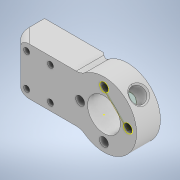
# Autodesk Inventor part: armtip_1
Saved by Autodesk Inventor 2020 (Build 240168000, 168)
## iProperties
Created: 2019-10-15
Part Number: armtip_1
Material: Generic
Document SubType Name: Modeling
Designer: psrob
Density: 1 g/cm^3
Appearance: Default
Author: psrob
Autodesk Inventor part; units mm, degrees
ref_plane "YZ Plane" through (0, 0, 0) normal (1, 0, 0) x (0, 1, 0)
ref_plane "XZ Plane" through (0, 0, 0) normal (0, 1, 0) x (-1, 0, 0)
ref_plane "XY Plane" through (0, 0, 0) normal (0, 0, 1) x (1, 0, 0)
sketch "Sketch1" plane through (0, 0, 0) normal (0, 0, 1) x (1, 0, 0)
  circle A0 centre (0, 0) radius 11 projected
  circle A1 centre (0, 0) radius 5 projected
  circle A2 centre (0, 0) radius 5.5
  circle A3 centre (0, 0) radius 11
  point P0 (0, 0)
  dimension "d0" = 11
  dimension "d1" = 22
  constraints: 2 centre point, 2 coincident
  measures "d0" diameter of A2
  measures "d1" diameter of A3
extrude "Extrusion1" add sketch "Sketch1" along normal blind 8 contours A0
sketch "Sketch2" plane through (0, 0, 8) normal (0, 0, 1) x (1, 0, 0)
  circle A0 centre (0, 0) radius 11 projected
  circle A1 centre (0, 0) radius 5.5 projected
  line L0 (0, 0) -> (0, 8)
  circle A2 centre (0, 8) radius 1.5
  circle A3 centre (-8, 0) radius 1.5
  circle A4 centre (0, -8) radius 1.5
  circle A5 centre (8, 0) radius 1.5
  point P0 (0, 0)
  dimension "d4" = 8
  dimension "d5" = 3
  dimension "d8" = 360
  constraints: 4 centre point, 2 end point, 1 coincident, 1 vertical, 9 other
  measures "d4" distance of L0.start L0.end
  measures "d5" diameter of A2
extrude "Extrusion2" cut sketch "Sketch2" against normal blind 10 contours A2 | A3 | A4 | A5
sketch "Sketch3" plane through (0, 0, 8) normal (0, 0, 1) x (1, 0, 0)
  circle A0 centre (0, -8) radius 1.5 projected
  circle A1 centre (8, 0) radius 1.5 projected
  circle A2 centre (-8, 0) radius 1.5 projected
  circle A3 centre (0, 8) radius 1.5 projected
  circle A4 centre (0, 0) radius 11 projected
  circle A5 centre (0, 0) radius 5.5 projected
  line L0 (0, 0) -> (-30, 0)
  line L1 (-30, 0) -> (-15, 0)
  line L2 (-30, 0) -> (-30, 8)
  line L3 (-30, 0) -> (-30, -8)
  line L4 (-30, -8) -> (-7.5498, -8)
  circle A6 centre (0, 0) radius 11 projected
  line L5 (-30, 8) -> (-7.5498, 8)
  point P0 (0, 0)
  point P1 (-7.5498, -8)
  dimension "d12" = 30
  dimension "d13" = 15
  dimension "d14" = 8
  dimension "d15" = 8
  constraints: 12 end point, 2 perpendicular, 2 point on circle, 1 horizontal, 1 midpoint, 1 parallel, 1 vertical
  measures "d12" distance of L0.start L0.end
  measures "d13" distance of L0.end L1.end
  measures "d14" distance of L0.end L2.end
  measures "d15" distance of L0.end L3.end
extrude "Extrusion3" add sketch "Sketch3" against normal blind 10 contours A4 L0 L2 L5 | L4 L3 L0 A4
chamfer "Chamfer1" distance 2 angle 45 1 edges at (-11, 0, -2)
sketch "Sketch4" plane through (0, 0, -2) normal (0, 0, -1) x (-1, 0, 0)
  arc A0 (10.247, -8) -> (10.247, 8) centre (0, 0) ccw projected
  line L0 (10.247, -8) -> (30, -8) projected
  line L1 (30, -8) -> (30, 8) projected
  line L2 (30, 8) -> (10.247, 8) projected
  line L3 (15, -3) -> (15, 3)
  line L4 (15, 3) -> (45, 3)
  line L5 (45, 3) -> (45, -3)
  line L6 (45, -3) -> (15, -3)
  line L7 (15, -3) -> (45, 3) construction
  line L8 (15, 3) -> (45, -3) construction
  line L9 (30, -8) -> (30, 8) projected
  point P0 (0, 0)
  point P1 (30, 0)
  point P2 (30, -3)
  point P3 (30, 3)
  dimension "d21" = 6
  dimension "d22" = 30
  constraints: 12 end point, 3 midpoint, 2 parallel, 2 perpendicular
  measures "d21" distance of L3.start L3.end
  measures "d22" distance of L3.end L4.end
extrude "Extrusion4" cut sketch "Sketch4" against normal blind 3 contours L6 L3 L4 L1
sketch "Sketch5" plane through (0, 0, -2) normal (0, 0, -1) x (-1, 0, 0)
  line L0 (15, 3) -> (30, 3) projected
  line L1 (30, 3) -> (30, 8) projected
  line L2 (30, 8) -> (10.247, 8) projected
  arc A0 (10.247, -8) -> (10.247, 8) centre (0, 0) ccw projected
  line L3 (10.247, -8) -> (30, -8) projected
  line L4 (30, -8) -> (30, -3) projected
  line L5 (30, -3) -> (15, -3) projected
  line L6 (15, -3) -> (15, 3) projected
  line L7 (30, 3) -> (30, -3) projected
  line L8 (30, 0) -> (26, 0)
  line L9 (26, 0) -> (26, -5.5)
  circle A1 centre (26, -5.5) radius 1
  line L10 (26, 0) -> (26, 5.5)
  circle A2 centre (26, 5.5) radius 1
  line L11 (26, -5.5) -> (18, -5.5)
  line L12 (18, -5.5) -> (18, 5.5)
  line L13 (18, 5.5) -> (26, 5.5)
  line L14 (26, 5.5) -> (26, -5.5)
  circle A3 centre (18, -5.5) radius 1
  circle A4 centre (18, 5.5) radius 1
  point P0 (0, 0)
  dimension "d25" = 4
  dimension "d26" = 5.5
  dimension "d27" = 2
  dimension "d28" = 5.5
  dimension "d29" = 2
  dimension "d30" = 8
  dimension "d31" = 11
  dimension "d32" = 2
  dimension "d33" = 2
  constraints: 14 end point, 4 centre point, 4 coincident, 2 horizontal, 2 parallel, 2 perpendicular, 1 midpoint, 1 vertical
  measures "d25" distance of L8.start L8.end
  measures "d26" distance of L8.end L9.end
  measures "d27" diameter of A1
  measures "d28" distance of L8.end L10.end
  measures "d29" diameter of A2
  measures "d30" distance of L12.end L13.end
  measures "d31" distance of L11.end L12.end
  measures "d32" diameter of A3
  measures "d33" diameter of A4
extrude "Extrusion5" cut sketch "Sketch5" against normal blind 10 contours A4 L13 L12 | L12 L13 A4 | A2 L13 L10 | L10 L13 A2 | A3 L11 L12 | L12 L11 A3 | A1 L11 L9 | L9 L11 A1
fillet "Fillet1" radius 5 2 edges at (-7.5498, 8, 4) (-7.5498, -8, 4)
chamfer "Chamfer2" distance 2 angle 45 1 edges at (-30, 0, 8)
fillet "Fillet2" radius 2 2 edges at (-29, 8, 7) (-29, -8, 7)
sketch "Sketch6" plane through (0, 0, 0) normal (0, 0, -1) x (-1, 0, 0)
  circle A0 centre (0, 8) radius 1.5 projected
  circle A1 centre (-8, 0) radius 1.5 projected
  point P0 (0, 0)
sketch "Sketch7" plane through (0, 0, 8) normal (0, 0, 1) x (1, 0, 0)
  circle A0 centre (0, 8) radius 1.5 projected
  circle A1 centre (8, 0) radius 1.5 projected
  point P0 (0, 0)
ref_plane "Work Plane1" through (0, 8, 0) normal (-0.7071068, -0.7071068, 0) x (0.7071068, -0.7071068, 0)
sketch "Sketch8" plane through (0, 8, 0) normal (-0.7071068, -0.7071068, 0) x (0.7071068, -0.7071068, 0)
  line L0 (0.1569, 8) -> (0.1569, 0) projected
  line L1 (1.5, 8) -> (1.5, 0) projected
  line L2 (12.8137, 0) -> (9.8137, 0) projected
  line L3 (9.8137, 8) -> (12.8137, 8) projected
  line L4 (1.5, 0) -> (-1.5, 0) projected
  line L5 (-1.5, 8) -> (1.5, 8) projected
  line L6 (0.1569, 4) -> (11.1569, 4)
  line L7 (11.1569, 8) -> (11.1569, 0) projected
  circle A0 centre (5.6569, 4) radius 2.5
  point P0 (5.6569, 0)
  dimension "d41" = 5
  constraints: 3 midpoint, 2 end point, 1 centre point
  measures "d41" diameter of A0
extrude "Extrusion6" cut sketch "Sketch8" against normal mid plane 12 contours A0 L6 | L6 A0
chamfer "Chamfer3" distance 0.5 angle 45 1 edges at (5.8069, 9.3424, 3.9975)
body "Solid1"
